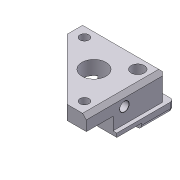
# Autodesk Inventor part: FOX-ME-121-03
Saved by Autodesk Inventor 2014 SP1 (Build 180222100, 222)
## iProperties
Created: 2011-09-07
Part Number: FOX-ME-121-03
Document SubType Name: Modeling
Designer: Robert Davis
Density: 2.71 g/cm^3
Material: Aluminum-6061
Mass: 4.06263 g
Surface Area: 12.1744 cm^2
Volume: 1.49912 cm^3
Description: RAIL END, -Z W/SPRING
Appearance: Aluminum - Flat
Author: Robert Davis
Autodesk Inventor part; units mm, degrees
ref_plane "YZ Plane" through (0, 0, 0) normal (1, 0, 0) x (0, 1, 0)
ref_plane "XZ Plane" through (0, 0, 0) normal (0, 1, 0) x (-1, 0, 0)
ref_plane "XY Plane" through (0, 0, 0) normal (0, 0, 1) x (1, 0, 0)
sketch "Sketch1" plane through (0, 0, 0) normal (0, 0, 1) x (1, 0, 0)
  line L0 (-4.25, 4.25) -> (4.25, 4.25)
  line L1 (4.25, 4.25) -> (4.25, -4.25)
  line L2 (4.25, -4.25) -> (-4.25, -4.25)
  line L3 (-4.25, -4.25) -> (-4.25, 4.25)
  point P0 (0, 0)
  dimension "d0" = 8.5
  dimension "d1" = 8.5
  dimension "d2" = 4.25
  dimension "d3" = 4.25
  constraints: 8 end point, 2 horizontal, 2 vertical
  measures "d0" distance of L0.start L0.end
  measures "d1" distance of L0.end L1.end
  measures "d2" distance from line of L0 point (0, 0)
  measures "d3" distance from line of L1 point (0, 0)
extrude "Extrusion1" add sketch "Sketch1" along normal blind 2.5
fillet "Fillet2" radius 1 3 edges at (4.25, 4.25, 1.25) (4.25, 0, 0) (0, 4.25, 0)
sketch "Sketch10" plane through (0, 0, 2.5) normal (0, 0, 1) x (1, 0, 0)
  line L0 (4.25, 3.25) -> (4.25, -4.25) projected
  line L1 (-4.25, 4.25) -> (3.25, 4.25) projected
  line L2 (3.25, 3.25) -> (-17.75, 3.25)
  line L3 (-17.75, 3.25) -> (-17.75, -17.75)
  line L4 (-17.75, -17.75) -> (3.25, -17.75)
  line L5 (3.25, -17.75) -> (3.25, 3.25)
  point P0 (0, 0)
  dimension "d113" = 1
  dimension "d114" = 1
  dimension "d115" = 21
  dimension "d116" = 21
  constraints: 8 end point
  measures "d113" distance between parallel lines of L0 L5
  measures "d114" distance between parallel lines of L2 L1
  measures "d115" distance of L2.start L2.end
  measures "d116" distance of L4.end L2.start
extrude "Extrusion8" add sketch "Sketch10" along normal blind 7
hole "Hole9" at (3.25, -7.75, 6.5) direction (-1, 0, 0) diameter 2.3876 depth 5 tip angle 118 countersink diameter 2.54 countersink angle 120
hole "Hole10" at (-7.75, 3.25, 6.5) direction (0, -1, 0) diameter 2.3876 depth 5 tip angle 118 countersink diameter 2.54 countersink angle 120
hole "Hole11" at (-6.25, -6.25, 9.5) direction (0, 0, -1) diameter 6.35 depth 5
sketch "Sketch11" plane through (0, 0, 2.5) normal (0, 0, -1) x (-1, 0, 0)
  line L0 (17.75, -17.75) -> (-3.25, -17.75) projected
  line L1 (17.75, 3.25) -> (17.75, -17.75) projected
  line L2 (4.25, 3.25) -> (17.75, 3.25) projected
  line L3 (10.75, 3.25) -> (17.75, 3.25)
  line L4 (17.75, 3.25) -> (17.75, -17.75)
  line L5 (17.75, -17.75) -> (-3.25, -17.75)
  line L6 (-3.25, -17.75) -> (-3.25, -10.75)
  line L7 (-3.25, -10.75) -> (0.75, -10.75)
  line L8 (0.75, -10.75) -> (10.75, -0.75)
  line L9 (10.75, -0.75) -> (10.75, 3.25)
  point P0 (0, 0)
  dimension "d146" = 14
  dimension "d158" = 4
  constraints: 14 end point, 3 horizontal, 3 perpendicular, 3 vertical, 1 point on line
  measures "d146" distance between parallel lines of L7 L2
  measures "d158" distance of L8.end L3.start
extrude "Extrusion9" cut sketch "Sketch11" against normal blind 3.325
hole "Hole12" at (-0.25, -14.75, 5.825) direction (0, 0, 1) diameter 2.3876 end through all countersink diameter 2.54 countersink angle 120
hole "Hole13" at (-14.75, -0.25, 5.825) direction (0, 0, 1) diameter 2.3876 end through all countersink diameter 2.54 countersink angle 120
chamfer "Chamfer3" distance 16 angle 45 1 edges at (-17.75, -17.75, 7.6625)
chamfer "Chamfer4" distance 1 angle 45 2 edges at (-7.25, 3.25, 9.5) (3.25, -7.25, 9.5)
sketch "Sketch15" plane through (0, 0, 2.5) normal (0, 0, 1) x (1, 0, 0)
  line L0 (-4.25, 3.25) -> (3.25, 3.25) projected
  line L1 (3.25, 3.25) -> (3.25, -4.25) projected
  line L2 (4.25, -4.25) -> (3.25, -4.25) projected
  line L3 (4.25, 3.25) -> (4.25, -4.25) projected
  arc A0 (4.25, 3.25) -> (3.25, 4.25) centre (3.25, 3.25) ccw projected
  line L4 (-4.25, 4.25) -> (3.25, 4.25) projected
  line L5 (-4.25, 3.25) -> (-4.25, 4.25) projected
  point P0 (0, 0)
extrude "Extrusion11" [suppressed]
chamfer "Chamfer6" distance 1 angle 45 1 edges at (3.25, 3.25, 5.5)
hole "Hole16" at (-0.5, -0.5, 0) direction (0, 0, 1) diameter 3.4544 end through all countersink diameter 4.064 countersink angle 120
sketch "Sketch16" plane through (0, 0, 2.5) normal (0, 0, -1) x (-1, 0, 0)
  line L0 (-3.25, -10.75) -> (0.75, -10.75) projected
  line L1 (10.75, -0.75) -> (10.75, 3.25) projected
  line L2 (4.25, 3.25) -> (10.75, 3.25) projected
  line L3 (4.25, -4.25) -> (4.25, 3.25) projected
  line L4 (-3.25, -4.25) -> (4.25, -4.25) projected
  line L5 (-3.25, -10.75) -> (-3.25, -4.25) projected
  line L6 (4.25, 4.25) -> (10.75, 4.25)
  line L7 (10.75, 4.25) -> (10.75, -0.75)
  line L8 (10.75, -0.75) -> (0.75, -10.75)
  line L9 (0.75, -10.75) -> (-4.25, -10.75)
  line L10 (-4.25, -10.75) -> (-4.25, -4.25)
  line L11 (-4.25, -4.25) -> (4.25, -4.25)
  line L12 (4.25, -4.25) -> (4.25, 4.25)
  point P0 (0, 0)
  dimension "d213" = 1
  dimension "d214" = 1
  constraints: 14 end point, 4 collinear, 2 parallel
  measures "d213" distance between parallel lines of L10 L5
  measures "d214" distance between parallel lines of L2 L6
extrude "Extrusion12" add sketch "Sketch16" along normal blind 1
body "Solid1"
